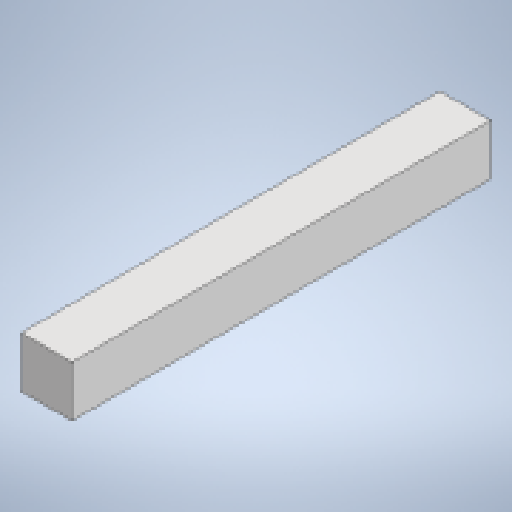
# Autodesk Inventor part: Refuerzo bisagra
Saved by Autodesk Inventor 2024 (Build 280153000, 153)
## iProperties
Created: 2025-03-01
Part Number: Refuerzo bisagra
Material: Genérico
Document SubType Name: Modeling
Designer: sergi
Density: 1 g/cm^3
Appearance: Valor por defecto
Author: sergi
Autodesk Inventor part; units mm, degrees
ref_plane "YZ Plane" through (0, 0, 0) normal (1, 0, 0) x (0, 1, 0)
ref_plane "XZ Plane" through (0, 0, 0) normal (0, 1, 0) x (-1, 0, 0)
sketch "Boceto1" plane through (0, 0, 0) normal (0, 1, 0) x (-1, 0, 0)
  line L0 (0, 0) -> (8, 0)
  line L1 (8, 0) -> (8, 66)
  line L2 (8, 66) -> (0, 66)
  line L3 (0, 66) -> (0, 0)
  dimension "d0" = 8
  dimension "d1" = 66
  constraints: 8 end point, 2 parallel, 1 horizontal, 1 perpendicular
  measures "d0" distance of L2.end L1.end
  measures "d1" distance of L1.end L0.end
extrude "Extrusión1" add sketch "Boceto1" along normal blind 8
ref_plane "Plano de trabajo1" through (-12.4, 18.08, 10) normal (0, 0, 1) x (1, 0, 0)
sketch "Boceto2" plane through (-12.4, 18.08, 10) normal (0, 0, 1) x (1, 0, 0)
  line L0 (4.4, -18.08) -> (12.4, -18.08) projected
  line L1 (12.4, -18.08) -> (12.4, -10.08) projected
  line L2 (4.4, -10.08) -> (12.4, -10.08) projected
  line L3 (4.4, -18.08) -> (4.4, -10.08) projected
  line L4 (8.4, -18.08) -> (8.4, -7.08)
  circle A0 centre (8.4, -14.08) radius 7
  line L5 (4.4, -18.08) -> (2.6554, -18.08)
  line L6 (4.4, -18.08) -> (14.1617, -18.0553)
  point P0 (12.4, -18.0597)
  dimension "d4" = 11
  constraints: 6 end point, 3 point on circle, 1 centre point, 1 horizontal, 1 midpoint, 1 point on line, 1 vertical
  measures "d4" distance of L4.start L4.end
ref_plane "Plano de trabajo2" through (-29.9, -16.92, 56) normal (0, 0, -1) x (0, 1, 0)
extrude "Extrusión2" add sketch "Boceto2" along normal up to surface (46 mm away) contours L6 L4 L0 | L5 A0 L4 L2 L3 | L3 L2 L4 L6 | L4 L6 L1 L0 | L4 L2 L1 L6 | L4 A0 L6 L1 L2
